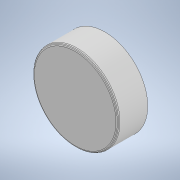
# Autodesk Inventor part: Base
Saved by Autodesk Inventor 2020 (Build 240168000, 168)
## iProperties
Created: 2020-02-27
Part Number: Base
Material: Generic
Document SubType Name: Modeling
Designer: othscs164
Density: 1 g/cm^3
Appearance: Default
Author: othscs164
Autodesk Inventor part; units mm, degrees
ref_plane "YZ Plane" through (0, 0, 0) normal (1, 0, 0) x (0, 1, 0)
ref_plane "XZ Plane" through (0, 0, 0) normal (0, 1, 0) x (-1, 0, 0)
ref_plane "XY Plane" through (0, 0, 0) normal (0, 0, 1) x (1, 0, 0)
sketch "Sketch1" plane through (0, 0, 0) normal (0, 0, 1) x (1, 0, 0)
  circle A0 centre (0, 0) radius 41.275
  circle A1 centre (0, 0) radius 47.625
  dimension "d0" = 82.55
  dimension "d1" = 6.35
  constraints: 2 centre point, 1 coincident
  measures "d0" diameter of A0
  measures "d1" radial gap between concentric circles of A0 A1
extrude "Extrusion1" add sketch "Sketch1" along normal blind 25.4
sketch "Sketch2" plane through (0, 0, 25.4) normal (0, 0, 1) x (1, 0, 0)
  circle A0 centre (0, 0) radius 47.625
  constraints: 1 centre point, 1 coincident
extrude "Extrusion2" add sketch "Sketch2" along normal blind 3.175
sketch "Sketch3" plane through (0, 0, 25.4) normal (0, 0, -1) x (-1, 0, 0)
  line L0 (11, 6) -> (-11, 6)
  line L1 (-11, 6) -> (-11, -6)
  line L2 (-11, -6) -> (11, -6)
  line L3 (11, -6) -> (11, 6)
  line L4 (11, 6) -> (-11, -6) construction
  line L5 (-11, 6) -> (11, -6) construction
  line L6 (-10.6662, 8.8412) -> (10.6662, 8.8412)
  line L7 (13.8412, 5.6662) -> (13.8412, -5.6662)
  line L8 (10.6662, -8.8412) -> (-10.6662, -8.8412)
  line L9 (-13.8412, -5.6662) -> (-13.8412, 5.6662)
  arc A0 (-10.6662, 8.8412) -> (-13.8412, 5.6662) centre (-10.6662, 5.6662) ccw
  arc A1 (-13.8412, -5.6662) -> (-10.6662, -8.8412) centre (-10.6662, -5.6662) ccw
  arc A2 (10.6662, -8.8412) -> (13.8412, -5.6662) centre (10.6662, -5.6662) ccw
  arc A3 (13.8412, 5.6662) -> (10.6662, 8.8412) centre (10.6662, 5.6662) ccw
  point P0 (0, 0)
  dimension "d6" = 22
  dimension "d7" = 12
  dimension "d8" = 3.175
  constraints: 20 end point, 8 point on circle, 8 tangent, 4 centre point, 4 parallel, 3 equal radius, 2 midpoint, 2 perpendicular, 1 horizontal, 3 other
  measures "d6" distance of L2.end L1.end
  measures "d7" distance of L1.end L0.end
  measures "d8" radius of A0
extrude "Extrusion3" add sketch "Sketch3" along normal blind 6.35
chamfer "Chamfer1" distance 1.5875 angle 45 8 edges at (0, 8.8412, 19.05) (12.9113, 7.9113, 19.05) (13.8412, 0, 19.05) (12.9113, -7.9113, 19.05) (0, -8.8412, 19.05) (-12.9113, -7.9113, 19.05) (-13.8412, 0, 19.05) (-12.9113, 7.9113, 19.05)
sketch "Sketch5" plane through (-13.8412, -5.6662, 25.4) normal (-1, 0, 0) x (0, 0, 1)
  line L0 (-0.1094, 0) -> (-8.0486, 0)
  line L1 (-8.0486, 0) -> (-8.0486, 11.3324)
  line L2 (-8.0486, 11.3324) -> (-0.1094, 11.3324)
  line L3 (-0.1094, 11.3324) -> (-0.1094, 0)
  point P0 (-25.4, 5.6662)
  constraints: 8 end point, 2 parallel, 1 horizontal, 1 perpendicular
extrude "Extrusion5" cut sketch "Sketch5" against normal blind 28.575
sketch "Sketch6" plane through (0, 0, 0) normal (0, 0, -1) x (-1, 0, 0)
  circle A0 centre (0, 0) radius 47.625 projected
  circle A1 centre (0, 0) radius 41.275 projected
extrude "Extrusion6" add sketch "Sketch6" along normal blind 4.5
chamfer "Chamfer2" distance 1.5875 angle 45 1 edges at (-47.625, 0, 28.575)
fillet "Fillet2" radius 1.5875 1 edges at (-46.0375, 0, 28.575)
fillet "Fillet3" radius 1.5875 1 edges at (-47.625, 0, 26.9875)
body "Solid1"
